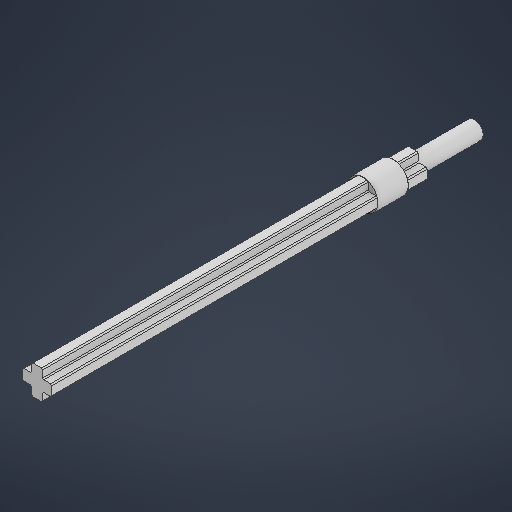
# Autodesk Inventor part: EjecilindroGarraSTD
Saved by Autodesk Inventor 2026.2 (Build 302298010, 298A)
## iProperties
Created: 2026-04-16
Part Number: EjecilindroGarraSTD
Material: Genérico
Document SubType Name: Modeling
Designer: Jose Carlos
Density: 1 g/cm^3
Appearance: Valor por defecto
Author: Jose Carlos
Autodesk Inventor part; units mm, degrees
ref_plane "Plano de trabajo1" through (0, 0, 0) normal (0, 0, 1) x (1, 0, 0)
sketch "Boceto1" plane through (0, 0, 0) normal (0, 0, 1) x (1, 0, 0)
  circle A0 centre (-10, -5) radius 1.4
  point P0 (0, 0)
  dimension "d0" = 2.8
  constraints: 1 centre point, 1 coincident
  measures "d0" diameter of A0
extrude "Extrusión1" add sketch "Boceto1" along normal blind 65 and the other way blind 7
sketch "Boceto3" plane through (-10, -5, 65) normal (0, 0, 1) x (1, 0, 0)
  line L0 (-2.4, 0.9) -> (2.4, 0.9)
  line L1 (2.4, 0.9) -> (2.4, -0.9)
  line L2 (2.4, -0.9) -> (-2.4, -0.9)
  line L3 (-2.4, -0.9) -> (-2.4, 0.9)
  line L4 (-2.4, 0.9) -> (2.4, -0.9) construction
  line L5 (2.4, 0.9) -> (-2.4, -0.9) construction
  circle A0 centre (0, 0) radius 1.4 projected
  line L6 (-0.9, 2.4) -> (0.9, 2.4)
  line L7 (0.9, 2.4) -> (0.9, -2.4)
  line L8 (0.9, -2.4) -> (-0.9, -2.4)
  line L9 (-0.9, -2.4) -> (-0.9, 2.4)
  line L10 (-0.9, 2.4) -> (0.9, -2.4) construction
  line L11 (0.9, 2.4) -> (-0.9, -2.4) construction
  point P0 (10, 5)
  point P1 (0.9, 0.9)
  point P2 (-0.9, 0.9)
  point P3 (-0.9, -0.9)
  point P4 (0.9, -0.9)
  dimension "d11" = 4.8
  dimension "d12" = 1.8
  constraints: 24 end point, 4 midpoint, 4 parallel, 4 perpendicular, 2 horizontal, 1 coincident
  measures "d11" distance of L0.start L0.end
  measures "d12" distance of L0.end L1.end
ref_plane "Plano de trabajo2" through (-27.5, -25, 0) normal (0, 0, 1) x (1, 0, 0)
ref_plane "Plano de trabajo4" through (-27.5, -25, 3.2373) normal (0, 0, 1) x (1, 0, 0)
extrude "Extrusión3" add sketch "Boceto3" against normal up to surface (61.7627 mm away) contours L0 A0 L2 L3 | L0 L9 L2 A0 | L9 A0 L7 L0 | L0 L7 L2 L9 | L9 L6 L7 A0 | L0 A0 L2 L7 | L2 L7 A0 L9 | A0 L7 L8 L9 | L0 L1 L2 A0
chamfer "Chaflán1" distance 0.2 angle 45 8 edges at (-7.6, -4.1, 34.1186) (-7.6, -5.9, 34.1186) (-9.1, -7.4, 34.1186) (-10.9, -7.4, 34.1186) (-12.4, -5.9, 34.1186) (-12.4, -4.1, 34.1186) (-10.9, -2.6, 34.1186) (-9.1, -2.6, 34.1186)
ref_plane "Plano de trabajo3" through (-10, -5, 3) normal (0, 0, 1) x (0, -1, 0)
ref_plane "Plano de trabajo5" through (-22.3692, -98.1544, 6.2373) normal (0, 0, 1) x (1, 0, 0)
ref_plane "Plano de trabajo6" through (-22.3692, -98.1544, 6.2373) normal (0, 0, 1) x (1, 0, 0)
ref_plane "Plano de trabajo7" through (-10, -5, 6.4373) normal (0, 0, 1) x (0, -1, 0)
sketch "Boceto4" plane through (-10, -5, 3) normal (0, 0, 1) x (0, -1, 0)
  circle A0 centre (0, 0) radius 2.5
  point P0 (-5, 10)
  point P1 (-1.2041, 2.1909)
  dimension "d20" = 5
  constraints: 1 coincident, 4 other
extrude "Extrusión4" add sketch "Boceto4" along normal blind 5 from surface at 3.4373
